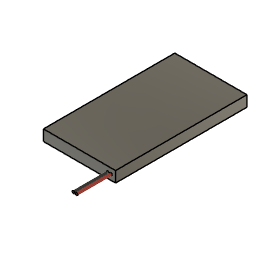
OpenBook+Final (Autodesk Fusion 360 archive; units mm, degrees)
design "Baterie_TSC v1"
Autodesk Fusion 360 part; units mm, degrees
box "BoxPrimitive1" add length 76.5 width 42 height 6.3 placed x (0, 1, 0) y (-1, 0, 0) z (0, 0, 1) at (42, 0, 0)
cylinder "CylinderPrimitive1" add diameter 1.5 height 20 placed x (1, 0, 0) y (0, 0, 1) z (0, -1, 0) at (39.3422, 0, 3.15)
cylinder "CylinderPrimitive2" add diameter 1.5 height 20 placed x (1, 0, 0) y (0, 0, 1) z (0, -1, 0) at (37.5, 0, 3.15)
